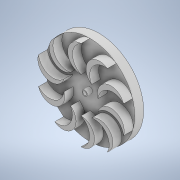
# Autodesk Inventor part: 20220701_fan_wing10
Saved by Autodesk Inventor 2020 (Build 240168000, 168)
## iProperties
Created: 2022-07-01
Part Number: 20220701_fan_wing10
Material: 一般
Document SubType Name: Modeling
Designer: Naggy
Density: 1 g/cm^3
Appearance: 既定
Author: Naggy
Autodesk Inventor part; units mm, degrees
ref_plane "YZ Plane" through (0, 0, 0) normal (1, 0, 0) x (0, 1, 0)
ref_plane "XZ Plane" through (0, 0, 0) normal (0, 1, 0) x (-1, 0, 0)
ref_plane "XY Plane" through (0, 0, 0) normal (0, 0, 1) x (1, 0, 0)
sketch "スケッチ1" plane through (0, 0, 0) normal (0, 0, 1) x (1, 0, 0)
  circle A0 centre (0, 0) radius 25
  dimension "d0" = 50
  constraints: 1 centre point, 1 coincident
  measures "d0" diameter of A0
extrude "押し出し1" add sketch "スケッチ1" along normal blind 5
sketch "スケッチ2" plane through (0, 0, 5) normal (0, 0, 1) x (1, 0, 0)
  circle A0 centre (0, 0) radius 10
  circle A1 centre (0, 0) radius 25 projected
  arc A2 (0, 25) -> (0, 10) centre (0, 17.5) ccw
  arc A3 (0, 25) -> (0, 10) centre (3.5, 17.5) ccw
  arc A4 (-14.6946, 20.2254) -> (-5.8779, 8.0902) centre (-10.2862, 14.1578) ccw
  arc A5 (-14.6946, 20.2254) -> (-5.8779, 8.0902) centre (-7.4547, 16.215) ccw
  arc A6 (-23.7764, 7.7254) -> (-9.5106, 3.0902) centre (-16.6435, 5.4078) ccw
  arc A7 (-23.7764, 7.7254) -> (-9.5106, 3.0902) centre (-15.5619, 8.7365) ccw
  arc A8 (-23.7764, -7.7254) -> (-9.5106, -3.0902) centre (-16.6435, -5.4078) ccw
  arc A9 (-23.7764, -7.7254) -> (-9.5106, -3.0902) centre (-17.725, -2.0791) ccw
  arc A10 (-14.6946, -20.2254) -> (-5.8779, -8.0902) centre (-10.2862, -14.1578) ccw
  arc A11 (-14.6946, -20.2254) -> (-5.8779, -8.0902) centre (-13.1178, -12.1005) ccw
  arc A12 (0, -25) -> (0, -10) centre (0, -17.5) ccw
  arc A13 (0, -25) -> (0, -10) centre (-3.5, -17.5) ccw
  arc A14 (14.6946, -20.2254) -> (5.8779, -8.0902) centre (10.2862, -14.1578) ccw
  arc A15 (14.6946, -20.2254) -> (5.8779, -8.0902) centre (7.4547, -16.215) ccw
  arc A16 (23.7764, -7.7254) -> (9.5106, -3.0902) centre (16.6435, -5.4078) ccw
  arc A17 (23.7764, -7.7254) -> (9.5106, -3.0902) centre (15.5619, -8.7365) ccw
  arc A18 (23.7764, 7.7254) -> (9.5106, 3.0902) centre (16.6435, 5.4078) ccw
  arc A19 (23.7764, 7.7254) -> (9.5106, 3.0902) centre (17.725, 2.0791) ccw
  arc A20 (14.6946, 20.2254) -> (5.8779, 8.0902) centre (10.2862, 14.1578) ccw
  arc A21 (14.6946, 20.2254) -> (5.8779, 8.0902) centre (13.1178, 12.1005) ccw
  dimension "d3" = 20
  dimension "d4" = 3.5
  dimension "d7" = 360
  constraints: 40 point on circle, 20 centre point, 2 vertical alignment, 1 coincident, 65 other
  measures "d4" distance of A3.centre A2.centre
extrude "押し出し2" add sketch "スケッチ2" along normal blind 5 contours A18 A19 | A16 A17 | A20 A21 | A14 A15 | A2 A3 | A12 A13 | A4 A5 | A10 A11 | A6 A7 | A8 A9
sketch "スケッチ3" plane through (0, 0, 5) normal (0, 0, 1) x (1, 0, 0)
  point P0 (0, 0)
  point P1 (0, 0)
  constraints: 1 coincident
hole "穴1" at (0, 0, 5) direction (0, 0, -1) diameter 2 depth 6 tip angle 118
sketch "スケッチ4" plane through (0, 0, 5) normal (0, 0, 1) x (1, 0, 0)
  circle A0 centre (0, 0) radius 1.5
  dimension "d18" = 3
  constraints: 1 centre point, 1 coincident
  measures "d18" diameter of A0
extrude "押し出し3" add sketch "スケッチ4" along normal blind 3
sketch "スケッチ5" plane through (0, 0, 8) normal (0, 0, 1) x (1, 0, 0)
  point P0 (0, 0)
  point P1 (0, 0)
  constraints: 1 coincident
hole "穴2" at (0, 0, 8) direction (0, 0, -1) diameter 2 depth 6 tip angle 118
sketch "スケッチ6" plane through (0, 0, 0) normal (1, 0, 0) x (0, 1, 0)
  point P0 (0, 0)
  point P1 (0, 6.0053)
hole "穴3" at (0, 0, 6.0053) direction (-1, 0, 0) diameter 1 depth 6 tip angle 118
